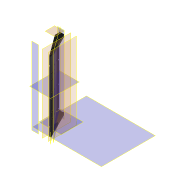
# Autodesk Inventor part: 40_ZTable_7Inch_Display_Housing_adjustable_dibondcompatible
Saved by Autodesk Inventor 2022 (Build 260153000, 153)
## iProperties
Created: 2023-03-04
Part Number: 40_ZTable_7Inch_Display_Housing_adjustable_dibondcompatible
Material: Generisch
Document SubType Name: Modeling
Designer: diederichbenedict
Density: 1 g/cm^3
Appearance: Glatt - Schwarz
Mass: 93.2551 g
Surface Area: 433.273 cm^2
Volume: 93.2551 cm^3
Author: diederichbenedict
Autodesk Inventor part; units mm, degrees
ref_plane "YZ Plane" through (0, 0, 0) normal (1, 0, 0) x (0, 1, 0)
ref_plane "XZ Plane" through (0, 0, 0) normal (0, 1, 0) x (-1, 0, 0)
ref_plane "Arbeitsebene1" through (15, 0, 0) normal (0, 0, -1) x (-1, 0, 0)
sketch "Skizze1" plane through (0, 0, 0) normal (0, 0, 1) x (1, 0, 0)
  line L0 (2, -17.5) -> (5, -17.5) projected
  line L1 (5, -9) -> (5, -17.5) projected
  arc A0 (9, -5) -> (5, -9) centre (9, -9) ccw projected
  line L2 (14.332, -5) -> (9, -5) projected
  line L3 (14.332, 0) -> (14.332, -5) projected
  line L4 (9, 0) -> (14.332, 0) projected
  arc A1 (9, 0) -> (0, -9) centre (9, -9) ccw projected
  line L5 (0, -156) -> (0, -9) projected
  arc A2 (0, -156) -> (9, -165) centre (9, -156) ccw projected
  line L6 (14.332, -165) -> (9, -165) projected
  line L7 (14.332, -160) -> (14.332, -165) projected
  line L8 (9, -160) -> (14.332, -160) projected
  arc A3 (5, -156) -> (9, -160) centre (9, -156) ccw projected
  line L9 (5, -147.5) -> (5, -156) projected
  line L10 (5, -147.5) -> (2, -147.5) projected
  line L11 (2, -147.5) -> (2, -117.5) projected
  line L12 (2, -117.5) -> (5, -117.5) projected
  line L13 (5, -97.5) -> (5, -117.5) projected
  line L14 (5, -97.5) -> (2, -97.5) projected
  line L15 (2, -97.5) -> (2, -67.5) projected
  line L16 (2, -67.5) -> (5, -67.5) projected
  line L17 (5, -47.5) -> (5, -67.5) projected
  line L18 (5, -47.5) -> (2, -47.5) projected
  line L19 (2, -47.5) -> (2, -17.5) projected
  circle A4 centre (7.5, -162.5) radius 1.6 projected
  circle A5 centre (2.5, -7.5) radius 1.6 projected
  circle A6 centre (2.5, -157.5) radius 1.6 projected
  circle A7 centre (7.5, -2.5) radius 1.6 projected
  circle A8 centre (2.5, -107.5) radius 1.6 projected
  circle A9 centre (2.5, -57.5) radius 1.6 projected
  arc A10 (-6, -156) -> (9, -171) centre (9, -156) ccw
  line L20 (-6, -156) -> (-6, -9)
  arc A11 (9, 6) -> (-6, -9) centre (9, -9) ccw
  line L21 (9, 6) -> (20.332, 6)
  line L22 (20.332, 6) -> (20.332, -11)
  line L23 (20.332, -11) -> (11, -11)
  line L24 (11, -11) -> (11, -23.5)
  line L25 (11, -23.5) -> (8, -23.5)
  line L26 (8, -23.5) -> (8, -41.5)
  line L27 (8, -41.5) -> (11, -41.5)
  line L28 (11, -41.5) -> (11, -73.5)
  line L29 (11, -73.5) -> (8, -73.5)
  line L30 (8, -73.5) -> (8, -91.5)
  line L31 (8, -91.5) -> (11, -91.5)
  line L32 (11, -91.5) -> (11, -123.5)
  line L33 (11, -123.5) -> (8, -123.5)
  line L34 (8, -123.5) -> (8, -141.5)
  line L35 (8, -141.5) -> (11, -141.5)
  line L36 (11, -141.5) -> (11, -154)
  line L37 (11, -154) -> (20.332, -154)
  line L38 (20.332, -154) -> (20.332, -171)
  line L39 (20.332, -171) -> (9, -171)
  line L40 (14.332, -165) -> (14.332, -171)
  line L41 (14.332, 0) -> (14.332, 6)
  line L42 (5, -17.5) -> (5, -47.5)
  line L43 (5, -67.5) -> (5, -97.5)
  line L44 (5, -117.5) -> (5, -147.5)
  point P0 (0, 0)
  dimension "d0" = 6
  constraints: 50 end point, 4 point on circle, 3 point on line, 2 centre point, 2 collinear, 2 vertical, 21 other
  measures "d0" radial gap between concentric circles of A2 A10
extrude "Extrusion1" add sketch "Skizze1" along normal blind 5 contours L19 L18 L17 L16 L15 L14 L13 L12 L11 L10 L9 A3 L8 L7 L6 A2 L5 A1 L4 L3 L2 A0 L1 L0 | L0 L42 L18 L19 | L43 L14 L15 L16 | L44 L10 L11 L12
ref_plane "Arbeitsebene2" through (156, -165, 55) normal (0, -1, 0) x (1, 0, 0)
sketch "Skizze2" plane through (156, -165, 55) normal (0, -1, 0) x (1, 0, 0)
  line L0 (-114, 0) -> (-141.668, -55) projected
  line L1 (0, 0) -> (-114, 0) projected
  line L2 (-150.1, -50) -> (-150.1, -55) projected
  line L3 (-155.1, -50) -> (-151.9, -50) projected
  line L4 (-114, 0) -> (-114.045, 0)
  line L5 (-197.1189, -89.3845) -> (-122.5426, -0.508) projected
  line L6 (-114, 0) -> (-114.045, 0)
  line L7 (-156, -50) -> (-141.668, -50)
  line L8 (-141.668, -50) -> (-141.668, -55)
  line L9 (-114, 7) -> (-114, 0)
  line L10 (-122.5426, -0.508) -> (-116.2427, 7)
  line L11 (-116.2427, 7) -> (-114, 7)
  line L12 (-114, 0) -> (-114.045, 0)
  line L13 (-114, 7) -> (-156, -50)
  line L14 (-156, -50) -> (-156, -50)
  line L15 (-156, -55) -> (-156, -50) projected
  line L16 (-110.9817, 6) -> (-114, 0)
  line L17 (-110.9817, 6) -> (-114.7368, 6)
  dimension "d40" = 0
  constraints: 24 end point, 5 horizontal, 1 collinear, 1 perpendicular, 1 point on line, 1 vertical, 4 other
  measures "d40" distance from line of L15 L13.end
ref_plane "Arbeitsebene3" through (9, 0, -60) normal (0, 1, 0) x (0, 0, 1)
extrude "Extrusion2" add sketch "Skizze2" against normal up to surface (165 mm away) contours L0 L8 L7 L3 L13 L17 L9 | L9 L17 L16
ref_plane "Arbeitsebene4" through (9.5, -158.3, 0) normal (0, -1, 0) x (-1, 0, 0)
sketch "Skizze3" plane through (9.5, -158.3, 0) normal (0, -1, 0) x (-1, 0, 0)
  line L0 (-45.8, -47.6) -> (-31.2283, -47.6) projected
  line L1 (-45.8, -8) -> (-45.8, -47.6) projected
  line L2 (-39.92, -8) -> (-45.8, -8) projected
  line L3 (-39.92, -42.1) -> (-39.92, -8) projected
  line L4 (-35.7511, -42.1) -> (-39.92, -42.1) projected
  line L5 (-7.1379, -8) -> (-35.7511, -42.1) projected
  line L6 (2, -8) -> (-7.1379, -8) projected
  line L7 (-31.2283, -47.6) -> (2, -8) projected
  line L8 (-4.832, 0) -> (-35.5183, -61) projected
  line L9 (-11.4292, -13.1143) -> (-8.5094, -7.31)
  line L10 (-7.1379, -8) -> (-8.5094, -7.31)
  line L11 (2, -8) -> (-45.8, -8)
  line L12 (-45.8, -8) -> (-45.8, 0)
  line L13 (-45.8, 0) -> (2, 0)
  line L14 (2, 0) -> (2, -8)
  line L15 (6.289, -6) -> (-8.0705, -6)
  line L16 (-8.0705, -6) -> (-36.6838, -40.1)
  line L17 (-36.6838, -40.1) -> (-37.92, -40.1)
  line L18 (-37.92, -40.1) -> (-37.92, -6)
  line L19 (-37.92, -6) -> (-47.8, -6)
  line L20 (-47.8, -6) -> (-47.8, -49.6)
  line L21 (-47.8, -49.6) -> (-30.2957, -49.6)
  line L22 (-30.2957, -49.6) -> (6.289, -6)
  line L23 (6.289, -6) -> (2, -6)
  line L24 (2, -6) -> (2, 0)
  line L25 (2, 0) -> (6.289, 0)
  line L26 (6.289, 0) -> (6.289, -6)
  line L27 (-47.8, -6) -> (-45.8, -6)
  line L28 (-45.8, -6) -> (-45.8, 0)
  line L29 (-45.8, 0) -> (-47.8, 0)
  line L30 (-47.8, 0) -> (-47.8, -6)
  point P0 (9.5, 0)
  point P1 (-32.5, -55)
  dimension "d38" = 8
  dimension "d39" = 2
  constraints: 44 end point, 6 parallel, 4 perpendicular, 3 horizontal, 3 point on line, 7 other
  measures "d38" distance between parallel lines of L13 L11
  measures "d39" distance between parallel lines of L7 L22
extrude "Extrusion3" cut sketch "Skizze3" against normal blind 152
hole "Bohrung1" at (19.7479, -53.36, 31.8007) at (19.7479, -61.3909, 31.8007) at (19.7479, -103.36, 31.8007) at (19.7479, -111.3909, 31.8007) direction (0.8050558, 0, -0.593199) diameter 2.8 depth 14 tip angle 118 counterbore diameter 6.5 counterbore depth 3
ref_plane "Arbeitsebene5" through (-2.5744, 0, 5) normal (0, 1, 0) x (1, 0, 0)
ref_plane "Arbeitsebene7" through (39.3806, -165, 55) normal (-0.7660444, 0, 0.6427876) x (0.6427876, 0, 0.7660444)
sketch "Skizze10" plane through (37.8203, -165, 56.3275) normal (-0.8050558, 0, 0.593199) x (0.593199, 0, 0.8050558)
  circle A0 centre (-4.2065, 161) radius 1.6 projected
  circle A1 centre (-4.2065, 4) radius 1.6 projected
  point P0 (-67.4458, 165)
hole "Bohrung3" at (35.325, -161, 52.9411) at (35.325, -4, 52.9411) direction (0.8050558, 0, -0.593199) diameter 2.8 end through all counterbore diameter 6.5 counterbore depth 3
ref_plane "Arbeitsebene9" through (47.6354, -165, 57.8476) normal (-0.8050558, 0, 0.593199) x (0.593199, 0, 0.8050558)
sketch "Skizze12" plane through (47.6354, -165, 57.8476) normal (-0.8050558, 0, 0.593199) x (0.593199, 0, 0.8050558)
  circle A0 centre (-4.5, 75.5) radius 1.4
  circle A1 centre (-4.5, 89.5) radius 1.4
  circle A2 centre (-4.5, 115.5) radius 1.4
  circle A3 centre (-4.5, 129.5) radius 1.4
  circle A4 centre (-4.5, 49.5) radius 1.4
  circle A5 centre (-4.5, 35.5) radius 1.4
  point P0 (-74.8278, 165)
  constraints: 6 centre point, 6 coincident, 12 other
hole "Bohrung4" at (44.966, -129.5, 54.2249) at (44.966, -115.5, 54.2249) at (44.966, -89.5, 54.2249) at (44.966, -75.5, 54.2249) at (44.966, -49.5, 54.2249) at (44.966, -35.5, 54.2249) direction (-0.8050558, 0, 0.593199) diameter 2.8 end through all counterbore diameter 6.5 counterbore depth 6
ref_plane "Arbeitsebene10" through (41.2632, -165, 61) normal (0.9999995, 0, 0.0009712) x (0, 1, 0)
ref_plane "Arbeitsebene11" through (0, 0, 60) normal (0, 0, -1) x (-1, 0, 0)
sketch "Skizze16" plane through (0, 0, 60) normal (0, 0, -1) x (-1, 0, 0)
  circle A0 centre (-32.4, -32.6) radius 6.5 projected
  circle A1 centre (-32.4, -82.6) radius 2.75 projected
  circle A2 centre (-32.45, -132.55) radius 6.5 projected
  point P0 (0, 0)
hole "Bohrung6" at (32.4, -32.6, 60) at (32.4, -82.6, 60) at (32.45, -132.55, 60) direction (0, 0, -1) diameter 2.8 end through all counterbore diameter 6.5 counterbore depth 15
sketch "Skizze17" plane through (42, -165, 62) normal (-0.8050558, 0, 0.593199) x (0.593199, 0, 0.8050558)
  line L0 (17.3974, 0) -> (-91.8512, 0) projected
  line L1 (-21.1165, 80.9861) -> (-21.1165, 83.8139) projected
  ellipse E0 centre (-16.1834, 82.4) end of major axis (-21.6622, 82.4) minor radius 3.25 (-21.1165, 80.9861) -> (-21.1165, 83.8139) ccw projected
  line L2 (-21.1165, 130.9861) -> (-21.1165, 133.8139) projected
  ellipse E1 centre (-16.1834, 132.4) end of major axis (-21.6622, 132.4) minor radius 3.25 (-21.1165, 130.9861) -> (-21.1165, 133.8139) ccw projected
  line L3 (-21.1165, 31.1446) -> (-21.1165, 33.7554) projected
  ellipse E2 centre (-16.0991, 32.45) end of major axis (-21.5779, 32.45) minor radius 3.25 (-21.1165, 31.1446) -> (-21.1165, 33.7554) ccw projected
  line L4 (-70.8025, 156) -> (-70.8025, 9) projected
  circle A0 centre (-37.512, 103.6091) radius 3.25 projected
  circle A1 centre (-37.512, 53.6091) radius 3.25 projected
  circle A2 centre (-37.512, 111.64) radius 3.25 projected
  circle A3 centre (-37.512, 61.64) radius 3.25 projected
  circle A4 centre (-11.2526, 161) radius 3.25 projected
  circle A5 centre (-11.2526, 4) radius 3.25 projected
  circle A6 centre (-4.5, 129.5) radius 1.4 projected
  circle A7 centre (-4.5, 89.5) radius 1.4 projected
  circle A8 centre (-4.5, 49.5) radius 1.4 projected
  circle A9 centre (-4.5, 35.5) radius 1.4 projected
  circle A10 centre (-4.5, 75.5) radius 1.4 projected
  circle A11 centre (-4.5, 115.5) radius 1.4 projected
  line L5 (-37.512, 173.2437) -> (-37.512, 147.7518) construction
  line L6 (-47.512, 173.2437) -> (-47.512, 147.7518)
  line L7 (-27.512, 147.7518) -> (-27.512, 173.2437)
  arc A12 (-27.512, 173.2437) -> (-47.512, 173.2437) centre (-37.512, 173.2437) ccw
  arc A13 (-47.512, 147.7518) -> (-27.512, 147.7518) centre (-37.512, 147.7518) ccw
  line L8 (-70.8025, 0) -> (-70.8025, 9) projected
  line L9 (-1.2421, 0) -> (-70.8025, 0) projected
  line L10 (-1.2421, 0) -> (-1.2421, 165) projected
  line L11 (-1.2421, 165) -> (-70.8025, 165) projected
  line L12 (-70.8025, 156) -> (-70.8025, 165) projected
  point P0 (-74.8278, 165)
  point P1 (-37.512, 160.4977)
  dimension "d72" = 20
  constraints: 8 end point, 4 point on circle, 4 tangent, 2 centre point, 1 midpoint, 1 parallel, 1 vertical, 3 other
  measures "d72" diameter of A13
extrude "Extrusion11" [suppressed]
ref_plane "Arbeitsebene12" through (27.7632, -165, 60.9869) normal (0.9999995, 0, 0.0009712) x (0, 1, 0)
sketch "Skizze18" plane through (27.7632, -165, 60.9869) normal (0.9999995, 0, 0.0009712) x (0, 1, 0)
  line L0 (0, 0) -> (165, 0) projected
  ellipse E0 centre (161, -3.5284) end of major axis (164.25, -3.5284) minor radius 0.0032 projected
  ellipse E1 centre (129.5, -2.6209) end of major axis (128.1, -2.6209) minor radius 1.1263 projected
  ellipse E2 centre (35.5, -2.6209) end of major axis (34.1, -2.6209) minor radius 1.1263 projected
  circle A0 centre (144.5, -2.6209) radius 1.4
  circle A1 centre (20.5, -2.6209) radius 1.4
  point P0 (165, -60.9599)
  dimension "d77" = 2.8
  dimension "d78" = 2.8
  dimension "d79" = 15
  dimension "d80" = 15
  constraints: 2 centre point, 2 other
  measures "d77" diameter of A0
  measures "d78" diameter of A1
  measures "d79" distance of A1.centre point (35.5, -2.621)
  measures "d80" distance of point (129.5, -2.621) A0.centre
hole "Bohrung7" at (27.7657, -20.5, 58.366) at (27.7657, -144.5, 58.366) direction (0.9999995, 0, 0.0009712) diameter 2.9 end through all counterbore diameter 6.5 counterbore depth 14
ref_plane "Arbeitsebene14" through (45.0183, -82.5, 61) normal (0, -1, 0) x (1, 0, 0)
mirror "Spiegeln1" [suppressed]
sketch "Skizze19" plane through (0, 0, 0) normal (0, 0, -1) x (-1, 0, 0)
  line L0 (-3.211, -58.9334) -> (-3.211, -106.0666) projected
  arc A0 (-3.211, -108.9334) -> (-3.211, -106.0666) centre (-2.5, -107.5) ccw projected
  line L1 (-3.211, -108.9334) -> (-3.211, -156.0666) projected
  arc A1 (-3.8856, -158.3) -> (-3.211, -156.0666) centre (-2.5, -157.5) ccw projected
  line L2 (-3.8856, -158.3) -> (-5.7274, -158.3) projected
  arc A2 (-9, -160) -> (-5.7274, -158.3) centre (-9, -156) ccw projected
  line L3 (-14.332, -160) -> (-9, -160) projected
  line L4 (-14.332, -165) -> (-14.332, -160) projected
  line L5 (-9, -165) -> (-14.332, -165) projected
  arc A3 (-9, -165) -> (0, -156) centre (-9, -156) ccw projected
  line L6 (0, -9) -> (0, -156) projected
  arc A4 (0, -9) -> (-9, 0) centre (-9, -9) ccw projected
  line L7 (-14.332, 0) -> (-9, 0) projected
  line L8 (-14.332, -5) -> (-14.332, 0) projected
  line L9 (-9, -5) -> (-14.332, -5) projected
  arc A5 (-6.0487, -6.3) -> (-9, -5) centre (-9, -9) ccw projected
  line L10 (-6.0487, -6.3) -> (-3.5583, -6.3) projected
  arc A6 (-3.211, -8.9334) -> (-3.5583, -6.3) centre (-2.5, -7.5) ccw projected
  line L11 (-3.211, -8.9334) -> (-3.211, -56.0666) projected
  arc A7 (-3.211, -58.9334) -> (-3.211, -56.0666) centre (-2.5, -57.5) ccw projected
  circle A8 centre (-7.5, -2.5) radius 1.6 projected
  circle A9 centre (-7.5, -162.5) radius 1.6 projected
  arc A10 (0, -9) -> (-9, 0) centre (-9, -9) ccw projected
  line L12 (0, -9) -> (0, 0) projected
  line L13 (0, 0) -> (-9, 0) projected
  arc A11 (-9, -165) -> (0, -156) centre (-9, -156) ccw projected
  line L14 (0, -165) -> (-9, -165) projected
  line L15 (0, -165) -> (0, -156) projected
  point P0 (0, 0)
  point P1 (-9, -165)
  point P2 (0, -156)
  point P3 (0, -9)
  point P4 (-9, 0)
extrude "Extrusion12" cut sketch "Skizze19" against normal through all contours L13 L12 A4 | A3 L15 L14 | A8 | A9
ref_plane "Arbeitsebene13" through (47, -82.5, 61) normal (0, -1, 0) x (1, 0, 0)
